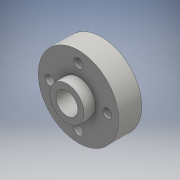
# Autodesk Inventor part: CouplingScrew
Saved by Autodesk Inventor 2016 (Build 200138000, 138)
## iProperties
Created: 2016-01-07
Part Number: CouplingScrew
Material: Generic
Document SubType Name: Modeling
Designer: m2memari
Density: 1 g/cm^3
Appearance: Default
Author: m2memari
Autodesk Inventor part; units mm, degrees
ref_plane "YZ Plane" through (0, 0, 0) normal (1, 0, 0) x (0, 1, 0)
ref_plane "XZ Plane" through (0, 0, 0) normal (0, 1, 0) x (-1, 0, 0)
ref_plane "XY Plane" through (0, 0, 0) normal (0, 0, 1) x (1, 0, 0)
sketch "Sketch1" plane through (0, 0, 0) normal (0, 1, 0) x (-1, 0, 0)
  circle A0 centre (0, 0) radius 3
  circle A1 centre (0, 0) radius 11.049
  circle A2 centre (0, -7.9375) radius 1.27
  circle A3 centre (7.9375, 0) radius 1.27
  circle A4 centre (0, 7.9375) radius 1.27
  circle A5 centre (-7.9375, 0) radius 1.27
  dimension "d4" = 6
  dimension "d6" = 22.098
  dimension "d10" = 2.54
  dimension "d11" = 7.9375
  dimension "d14" = 360
  constraints: 6 centre point, 2 coincident, 1 vertical alignment, 9 other
  measures "d4" diameter of A0
  measures "d6" diameter of A1
  measures "d10" diameter of A2
  measures "d11" distance of point (0, 0) A2.centre
extrude "Extrusion1" add sketch "Sketch1" along normal mid plane 6.35
sketch "Sketch2" plane through (0, 3.175, 0) normal (0, 1, 0) x (1, 0, 0)
  circle A0 centre (0, 0) radius 3
  circle A1 centre (0, 0) radius 4.699
  dimension "d18" = 6
  dimension "d19" = 9.398
  constraints: 2 centre point, 2 coincident
  measures "d18" diameter of A0
  measures "d19" diameter of A1
extrude "Extrusion2" add sketch "Sketch2" along normal blind 3.175
sketch "Sketch3" plane through (0, -3.175, 0) normal (0, -1, 0) x (1, 0, 0)
  circle A0 centre (0, 0) radius 3
  circle A1 centre (0, 0) radius 4.699
  dimension "d22" = 6
  dimension "d23" = 9.398
  constraints: 2 centre point, 2 coincident
  measures "d22" diameter of A0
  measures "d23" diameter of A1
extrude "Extrusion3" add sketch "Sketch3" along normal blind 3.175
body "Solid1"
